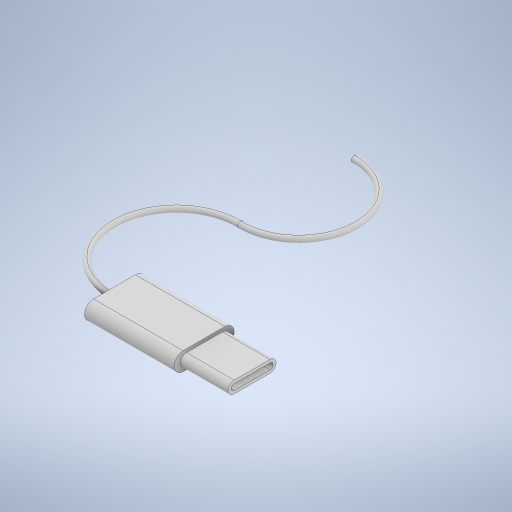
# Autodesk Inventor part: ctype charger
Saved by Autodesk Inventor 2024.3 (Build 283343000, 343)
## iProperties
Created: 2024-08-06
Part Number: ctype charger
Material: 일반
Document SubType Name: Modeling
Designer: naru4
Density: 1 g/cm^3
Appearance: 기본값
Author: naru4
Autodesk Inventor part; units mm, degrees
ref_plane "YZ Plane" through (0, 0, 0) normal (1, 0, 0) x (0, 1, 0)
ref_plane "XZ Plane" through (0, 0, 0) normal (0, 1, 0) x (-1, 0, 0)
ref_plane "XY Plane" through (0, 0, 0) normal (0, 0, 1) x (1, 0, 0)
sketch "스케치1" plane through (0, 0, 0) normal (0, 1, 0) x (-1, 0, 0)
  arc A0 (0.0028, -21.0994) -> (0, 0) centre (0.2331, -10.5497) ccw
  arc A1 (0.0028, -21.0994) -> (0, -40.0782) centre (-0.2043, -30.5888) ccw
  constraints: 4 point on circle, 2 centre point, 1 tangent
sketch "스케치2" plane through (0, 0, 0) normal (1, 0, 0) x (0, 1, 0)
  circle A0 centre (0, 0) radius 0.5
  dimension "d0" = 1
  constraints: 1 centre point, 1 coincident
  measures "d0" diameter of A0
sweep "스윕1" add profiles "스케치2" path "스케치1"
sketch "스케치3" plane through (0, 0, 0) normal (1, 0, 0) x (0, 0, -1)
  arc A0 (-3.5, 1.5) -> (-3.5, -1.5) centre (-3.5, 0) ccw
  arc A1 (3.5, -1.5) -> (3.5, 1.5) centre (3.5, 0) ccw
  line L0 (-3.5, 1.5) -> (3.5, 1.5)
  line L1 (-3.5, -1.5) -> (3.5, -1.5)
  point P0 (0, 0)
  dimension "d6" = 3
  dimension "d7" = 3
  constraints: 4 end point, 4 point on circle, 2 centre point, 1 horizontal, 1 parallel, 1 tangent
  measures "d6" diameter of A0
  measures "d7" diameter of A1
extrude "돌출1" add sketch "스케치3" along normal blind 15
sketch "스케치4" plane through (15, 0, 0) normal (1, 0, 0) x (0, 0, -1)
  arc A0 (-3, 1) -> (-3, -1) centre (-3, 0) ccw
  arc A1 (3, -1) -> (3, 1) centre (3, 0) ccw
  line L0 (-3, 1) -> (3, 1)
  line L1 (-3, -1) -> (3, -1)
  point P0 (0, 0)
  constraints: 4 end point, 4 point on circle, 2 centre point, 1 horizontal, 1 tangent
extrude "돌출2" add sketch "스케치4" along normal blind 8
sketch "스케치5" plane through (23, 0, 0) normal (1, 0, 0) x (0, 0, -1)
  arc A0 (-3, 0.5) -> (-3, -0.5) centre (-3, 0) ccw
  arc A1 (3, -0.5) -> (3, 0.5) centre (3, 0) ccw
  line L0 (-0.0026, 0.5) -> (21.1019, 0.5) projected
  line L1 (-3, 0.5) -> (3, 0.5)
  line L2 (-3, -0.5) -> (3, -0.5)
  point P0 (0, 0.5)
  point P1 (0, 0)
  point P2 (21.0994, 0.5)
  constraints: 4 end point, 4 point on circle, 2 centre point, 2 tangent, 1 point on line
extrude "돌출3" cut sketch "스케치5" against normal blind 8
